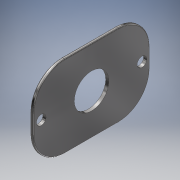
# Autodesk Inventor part: Component 7 (Cover Plate)
Saved by Autodesk Inventor 2018 (Build 220112000, 112)
## iProperties
Created: 2023-03-14
Part Number: Component 7 (Cover Plate)
Material: Generic
Document SubType Name: Modeling
Designer: Habib Mohamed
Density: 1 g/cm^3
Appearance: Semi-Polished
Author: Habib Mohamed
Autodesk Inventor part; units mm, degrees
ref_plane "YZ Plane" through (0, 0, 0) normal (1, 0, 0) x (0, 1, 0)
ref_plane "XZ Plane" through (0, 0, 0) normal (0, 1, 0) x (-1, 0, 0)
ref_plane "XY Plane" through (0, 0, 0) normal (0, 0, 1) x (1, 0, 0)
sketch "Sketch1" plane through (0, 0, 0) normal (1, 0, 0) x (0, 1, 0)
  circle A0 centre (0, 0) radius 5.5
  line L0 (3, 18.5) -> (-3, 18.5)
  line L1 (-13, 8.5) -> (-13, -8.5)
  line L2 (-3, -18.5) -> (3, -18.5)
  line L3 (13, -8.5) -> (13, 8.5)
  line L4 (13, 18.5) -> (-13, -18.5) construction
  line L5 (-13, 18.5) -> (13, -18.5) construction
  circle A1 centre (0, 16) radius 1.55
  line L6 (0, 0) -> (10.4906, 0) construction
  circle A2 centre (0, -16) radius 1.55
  line L7 (0, 0) -> (0, 32) construction
  arc A3 (13, 8.5) -> (3, 18.5) centre (3, 8.5) ccw
  arc A4 (-3, 18.5) -> (-13, 8.5) centre (-3, 8.5) ccw
  arc A5 (-13, -8.5) -> (-3, -18.5) centre (-3, -8.5) ccw
  arc A6 (3, -18.5) -> (13, -8.5) centre (3, -8.5) ccw
  dimension "d0" = 11
  dimension "d1" = 2.5
  dimension "d2" = 37
  dimension "d3" = 26
  dimension "d4" = 3.1
  dimension "d5" = 10
  constraints: 16 end point, 8 point on circle, 8 point on line, 8 tangent, 7 centre point, 3 equal radius, 3 midpoint, 2 coincident, 2 horizontal, 2 parallel, 1 perpendicular, 1 symmetric about line, 1 vertical, 1 other
  measures "d0" diameter of A0
  measures "d1" distance from line of A1.centre L0
  measures "d2" distance of L5.end L4.start
  measures "d3" distance of L4.start L5.start
  measures "d4" diameter of A1
  measures "d5" radius of A3
extrude "Extrusion1" add sketch "Sketch1" along normal blind 1
fillet "Fillet1" radius 0.25 16 edges at (1, 0, 18.5) (1, -10.0711, 15.5711) (1, -13, 0) (1, -10.0711, -15.5711) (1, 0, -18.5) (1, 10.0711, -15.5711) (1, 13, 0) (1, 10.0711, 15.5711) (0, 0, 18.5) (0, -10.0711, 15.5711) (0, -13, 0) (0, -10.0711, -15.5711) (0, 0, -18.5) (0, 10.0711, -15.5711) (0, 13, 0) (0, 10.0711, 15.5711)
body "Solid1"
